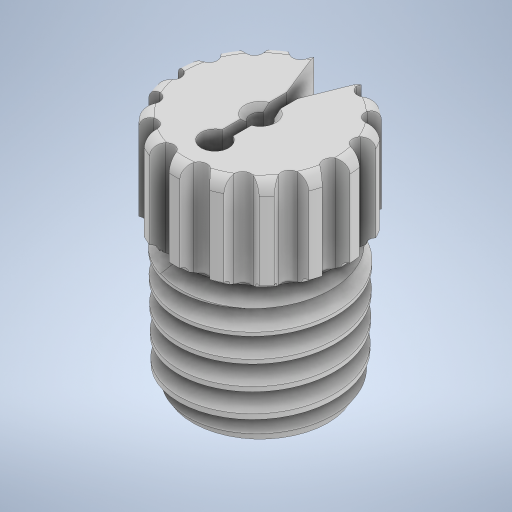
# Autodesk Inventor part: Ferula FO Cententelladores
Saved by Autodesk Inventor 2024.2 (Build 282272000, 272)
## iProperties
Created: 2025-08-12
Part Number: Ferula FO Cententelladores
Material: Generic
Document SubType Name: Modeling
Designer: ja.restrepo1
Density: 1 g/cm^3
Appearance: Default
Author: ja.restrepo1
Autodesk Inventor part; units mm, degrees
ref_plane "YZ Plane" through (0, 0, 0) normal (1, 0, 0) x (0, 1, 0)
ref_plane "XZ Plane" through (0, 0, 0) normal (0, 1, 0) x (-1, 0, 0)
ref_plane "XY Plane" through (0, 0, 0) normal (0, 0, 1) x (1, 0, 0)
sketch "Sketch1" plane through (0, 0, 0) normal (1, 0, 0) x (0, 1, 0)
  line L0 (8.1, 0.725) -> (-1.5, 0.725)
  line L1 (-1.5, 0.725) -> (-8.0042, 1.8719)
  line L2 (-8.5, 2.4627) -> (-8.5, 4.9025)
  line L3 (-7.3002, 5.6235) -> (0.293, 5.756)
  line L4 (2.1, 6.25) -> (7.7, 6.25)
  line L5 (8.5, 5.45) -> (8.5, 1.125)
  line L6 (8.5, 0) -> (-8.5, 0) construction
  line L7 (2.1, 6.25) -> (2.1, 6.1806)
  arc A0 (1.707, 5.7807) -> (2.1, 6.1806) centre (1.7, 6.1806) ccw
  line L8 (-7.3002, 5.6235) -> (-8.5, 4.9025)
  line L9 (8.5, 1.125) -> (8.1, 0.725)
  arc A1 (8.5, 5.45) -> (7.7, 6.25) centre (7.7, 5.45) ccw
  arc A2 (-8.5, 2.4627) -> (-8.0042, 1.8719) centre (-7.9, 2.4627) ccw
  line L10 (0.293, 5.756) -> (1.707, 5.7807) construction
  line L11 (1.707, 5.7807) -> (1.0244, 4.3683)
  line L12 (1.0244, 4.3683) -> (0.293, 5.756)
  point P0 (0, 0)
  point P1 (8.5, 0.725)
  point P2 (-8.5, 1.9593)
  point P3 (-8.5, 5.6025)
  point P4 (8.5, 6.25)
  point P5 (0, 0)
  point P6 (-8.5, 3.6826)
  point P7 (1, 5.7683)
  dimension "d0" = 17
  dimension "d1" = 10
  dimension "d2" = 6.4
  dimension "d3" = 10.6
  dimension "d4" = 170
  dimension "d5" = 91
  dimension "d6" = 0.725
  dimension "d7" = 6.25
  dimension "d8" = 5.75
  dimension "d9" = 0.4
  dimension "d11" = 1.2
  dimension "d12" = 0.7
  dimension "d13" = 0.4
  dimension "d14" = 45
  dimension "d15" = 0.8
  dimension "d16" = 0.6
  dimension "d43" = 9.5
  dimension "d44" = 1.4
  constraints: 27 end point, 9 point on line, 7 tangent, 6 point on circle, 3 centre point, 3 midpoint, 2 coincident, 2 horizontal, 2 perpendicular, 1 equal length, 1 parallel, 1 vertical, 1 vertical alignment
  measures "d0" distance of L6.start L6.end
  measures "d1" distance of point (8.5, 0.725) L0.end
  measures "d2" distance of L4.start point (8.5, 6.25)
  measures "d3" distance from line of L4.start L2
  measures "d4" angle of L1 L0
  measures "d5" angle of L2 L3
  measures "d6" distance from line of L0 point (0, 0)
  measures "d7" distance from line of point (0, 0) L4
  measures "d8" distance from line of point (0, 0) L3
  measures "d9" radius of A0
  measures "d11" distance of L3.start point (-8.5, 5.603)
  measures "d12" distance of L2.end point (-8.5, 5.603)
  measures "d13" distance of L5.end point (8.5, 0.725)
  measures "d14" angle of L5 L9
  measures "d15" radius of A1
  measures "d16" radius of A2
  measures "d43" distance from line of point (1, 5.768) L2
  measures "d44" vertical distance of L11.end point (1, 5.768)
revolve "Revolution2" add sketch "Sketch1" angle 360 about axis through (0, 8.5, 0) along (0, -1, 0)
sketch "Sketch3" plane through (0, 0, 0) normal (1, 0, 0) x (0, 1, 0)
  line L0 (-9.4, 0) -> (-9.4, 5.5) construction
  line L1 (0.293, 5.756) -> (0.293, -5.756) construction
  line L2 (0.293, 5.756) -> (-9.4, 5.756) construction
  line L3 (-9.4, 4.442) -> (-10.1586, 5.756)
  line L4 (-10.1586, 5.756) -> (-8.6414, 5.756)
  line L5 (-8.6414, 5.756) -> (-9.4, 4.442)
  point P0 (0, 0)
  point P1 (-9.4, 2.75)
  point P2 (-9.4, 5.318)
  dimension "d32" = 5.5
  dimension "d33" = 9.4
  dimension "d34" = 1.5172
  constraints: 10 end point, 2 horizontal, 2 vertical alignment, 1 collinear, 1 horizontal alignment, 1 midpoint, 1 vertical, 7 other
  measures "d32" distance of L0.start L0.end
  measures "d33" distance from line of point (0, 0) L0
  measures "d34" distance of L3.end L4.end
coil "Coil2" sketch "Sketch3" operation cut axis through (0, -10, 0) along (0, 1, 0) pitch 1.75 turns 5.95 hand right
sketch "Sketch4" plane through (0, 8.5, 0) normal (0, 1, 0) x (1, 0, 0)
  line L0 (-0.5196, 5.4953) -> (-1, 6.3274)
  line L1 (-1, 6.3274) -> (1, 6.3274)
  line L2 (1, 6.3274) -> (0.5196, 5.4953)
  arc A0 (-0.5196, 5.4953) -> (0.5196, 5.4953) centre (0, 5.7953) ccw
  point P0 (0, 0)
  point P1 (0, 5.75)
  point P2 (0, 4.5953)
  dimension "d45" = 5.75
  dimension "d46" = 2
  dimension "d47" = 0.6
  constraints: 6 end point, 2 point on circle, 2 point on line, 2 tangent, 1 centre point, 1 horizontal, 1 vertical alignment, 7 other
  measures "d45" distance of point (0, 0) point (0, 5.75)
  measures "d46" distance of L0.end L1.end
  measures "d47" radius of A0
extrude "agarre" cut sketch "Sketch4" against normal blind 7
pattern_circular "Circular Pattern1" count 15 over 360 about axis through (0, 7.7, 0) along (0, -1, 0) of "agarre"
sketch "Sketch6" plane through (0, 8.5, -5.7953) normal (0, 1, 0) x (1, 0, 0)
  arc A0 (-0.4, -8.1788) -> (0.4, -8.1788) centre (0, -9.0953) ccw
  line L0 (-0.4, -8.1788) -> (-0.4, -3.4788)
  line L1 (-0.4, -3.4788) -> (-2, 0.5212)
  line L2 (-2, 0.5212) -> (2, 0.5212)
  line L3 (2, 0.5212) -> (0.4, -3.4788)
  line L4 (0.4, -3.4788) -> (0.4, -8.1788)
  arc A1 (0.4, -8.1788) -> (-0.4, -8.1788) centre (0, -9.0953) ccw construction
  point P0 (0, -5.7953)
  point P1 (0, 0.5212)
  dimension "d53" = 2
  dimension "d54" = 3.3
  dimension "d55" = 0.8
  dimension "d56" = 4
  dimension "d57" = 4
  dimension "d58" = 4.7
  constraints: 10 end point, 4 point on circle, 2 centre point, 2 vertical alignment, 1 equal length, 1 horizontal alignment, 1 midpoint, 1 parallel, 1 perpendicular, 1 vertical
  measures "d53" diameter of A0
  measures "d54" distance of A0.centre point (0, -5.795)
  measures "d55" distance between parallel lines of L0 L4
  measures "d56" distance from line of L3.end L2
  measures "d57" distance of L1.end L2.end
  measures "d58" distance of L3.end L4.end
extrude "Extrusion2" cut sketch "Sketch6" against normal through all
body "Solid2"
